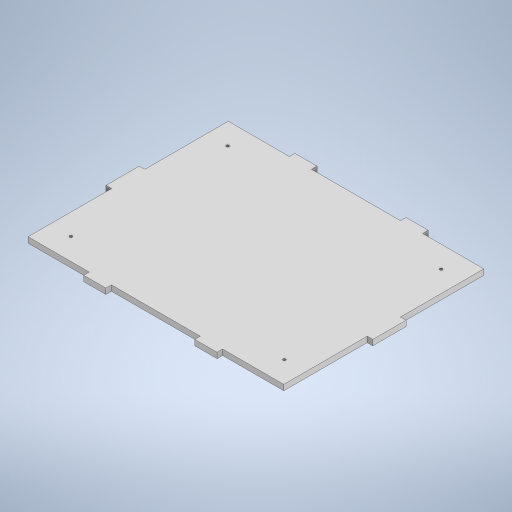
# Autodesk Inventor part: onderkant
Saved by Autodesk Inventor 2023 (Build 270158000, 158)
## iProperties
Created: 2023-06-01
Part Number: onderkant
Material: Generic
Document SubType Name: Modeling
Designer: Prestige
Density: 1 g/cm^3
Appearance: Default
Author: Prestige
Autodesk Inventor part; units mm, degrees
ref_plane "YZ Plane" through (0, 0, 0) normal (1, 0, 0) x (0, 1, 0)
ref_plane "XZ Plane" through (0, 0, 0) normal (0, 1, 0) x (-1, 0, 0)
ref_plane "XY Plane" through (0, 0, 0) normal (0, 0, 1) x (1, 0, 0)
sketch "Sketch1" plane through (0, 0, 0) normal (0, 1, 0) x (-1, 0, 0)
  line L0 (0, 0) -> (230, 0)
  line L1 (230, 0) -> (230, -180)
  line L2 (230, -180) -> (0, -180)
  line L3 (0, -180) -> (0, 0)
  dimension "d0" = 180
  dimension "d1" = 230
  constraints: 8 end point, 2 parallel, 1 horizontal, 1 perpendicular
  measures "d0" distance of L2.end L0.start
  measures "d1" distance between parallel lines of L3 L1
extrude "Extrusion1" add sketch "Sketch1" along normal blind 5
sketch "Sketch2" plane through (0, 0, -180) normal (0, 0, -1) x (-1, 0, 0)
  line L0 (0, 5) -> (230, 5) projected
  line L1 (55, 5) -> (75, 5)
  line L2 (75, 5) -> (75, 0)
  line L3 (75, 0) -> (55, 0)
  line L4 (55, 0) -> (55, 5)
  line L5 (0, 0) -> (230, 0) projected
  line L6 (155, 5) -> (175, 5)
  line L7 (175, 5) -> (175, 0)
  line L8 (175, 0) -> (155, 0)
  line L9 (155, 0) -> (155, 5)
  line L10 (0, 0) -> (0, 5) projected
  line L11 (230, 0) -> (230, 5) projected
  point P0 (175, 2.5)
  point P1 (155, 2.5)
  point P2 (230, 2.5)
  dimension "d4" = 20
  dimension "d5" = 20
  dimension "d6" = 80
  dimension "d7" = 55
  dimension "d8" = 55
  constraints: 16 end point, 4 parallel, 3 midpoint, 3 point on line, 2 horizontal, 2 perpendicular
  measures "d4" distance of point (175, 2.5) point (155, 2.5)
  measures "d5" distance between parallel lines of L4 L2
  measures "d6" distance between parallel lines of L2 L9
  measures "d7" distance between parallel lines of L10 L4
  measures "d8" distance of point (175, 2.5) point (230, 2.5)
extrude "Extrusion2" add sketch "Sketch2" along normal blind 5 and the other way blind 185 contours L0 L2 L3 L4 | L0 L7 L5 L9
sketch "Sketch3" plane through (0, 0, 0) normal (1, 0, 0) x (0, 0, -1)
  line L0 (0, 5) -> (180, 5) projected
  line L1 (0, 0) -> (180, 0) projected
  line L2 (75, 5) -> (105, 5)
  line L3 (105, 5) -> (105, 0)
  line L4 (105, 0) -> (75, 0)
  line L5 (75, 0) -> (75, 5)
  line L6 (180, 0) -> (180, 5) projected
  point P0 (180, 2.5)
  dimension "d13" = 30
  dimension "d14" = 75
  constraints: 8 end point, 2 parallel, 2 point on line, 1 horizontal, 1 midpoint, 1 perpendicular
  measures "d13" distance between parallel lines of L3 L5
  measures "d14" distance from line of point (180, 2.5) L3
extrude "Extrusion3" add sketch "Sketch3" along normal blind 5 and the other way blind 235 contours L0 L3 L1 L5
sketch "Sketch4" plane through (0, 5, 0) normal (0, 1, 0) x (1, 0, 0)
  line L0 (-230, 75) -> (-230, 0) projected
  line L1 (0, 180) -> (-55, 180) projected
  point P0 (0, 0)
  point P1 (-211, 160.5)
  point P2 (-19, 160.5)
  point P3 (-19, 19.5)
  point P4 (-211, 19.5)
  point P5 (-230, 37.5)
  dimension "d19" = 141
  dimension "d20" = 192
  dimension "d21" = 19
  dimension "d22" = 141
  dimension "d23" = 0
  dimension "d24" = 19.5
  constraints: 1 midpoint
  measures "d19" distance of point (-211, 19.5) point (-211, 160.5)
  measures "d20" distance of point (-211, 19.5) point (-19, 19.5)
  measures "d21" horizontal distance of point (-230, 37.5) point (-211, 19.5)
  measures "d22" distance of point (-19, 19.5) point (-19, 160.5)
  measures "d23" horizontal distance of point (-19, 160.5) point (-19, 19.5)
  measures "d24" distance from line of L1 point (-19, 160.5)
hole "Hole1" at (-211, 5, -160.5) at (-19, 5, -160.5) at (-19, 5, -19.5) at (-211, 5, -19.5) direction (0, -1, 0) diameter 2.459 end through all thread size "M3x0.5" class "6H" standard "ANSI Metric M Profile"
body "Solid1"
